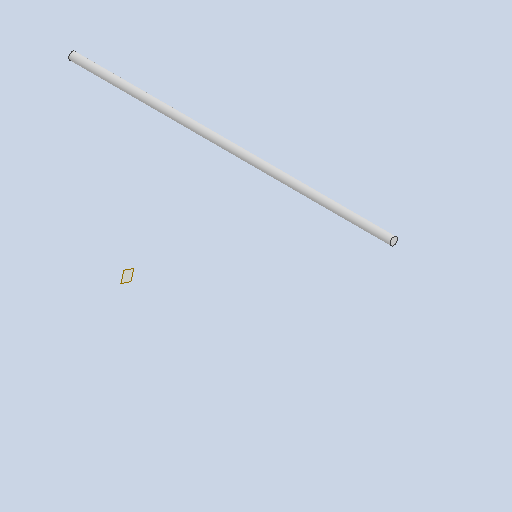
# Autodesk Inventor part: 12MM_X_AXIS_SHAFT
Saved by Autodesk Inventor 2025.2 (Build 292293000, 293)
## iProperties
Created: 2026-02-05
Part Number: 12MM_X_AXIS_SHAFT
Material: Generic
Document SubType Name: Modeling
Designer: composite
Density: 1 g/cm^3
Appearance: Default
Author: composite
Autodesk Inventor part; units mm, degrees
ref_plane "YZ Plane" through (0, 0, 0) normal (1, 0, 0) x (0, 1, 0)
ref_plane "XZ Plane" through (0, 0, 0) normal (0, 1, 0) x (-1, 0, 0)
ref_plane "XY Plane" through (0, 0, 0) normal (0, 0, 1) x (1, 0, 0)
sketch "Sketch1" plane through (0, 0, 0) normal (1, 0, 0) x (0, 1, 0)
  circle A0 centre (0, 0) radius 6
  dimension "d0" = 12
  constraints: 1 centre point, 1 coincident
  measures "d0" diameter of A0
extrude "Extrusion1" add sketch "Sketch1" along normal blind 10
sketch "Sketch2" plane through (0, 0, 0) normal (-1, 0, 0) x (0, 0, 1)
  circle A0 centre (0, 0) radius 6 projected
ref_plane "Work Plane1" through (-497, -256, -240) normal (-1, 0, 0) x (0, 0, 1)
ref_plane "Work Plane2" through (-697, -256, -240) normal (-1, 0, 0) x (0, 0, 1)
ref_plane "Work Plane3" through (-497, -256, -240) normal (-1, 0, 0) x (0, 0, 1)
ref_plane "Work Plane5" through (-481.5, -427.3957, -227.227) normal (1, 0, 0) x (0, 0.3162278, 0.9486833)
extrude "Extrusion3" add sketch "Sketch2" along normal up to surface (481.5 mm away)
sketch "Sketch3" plane through (-481.5, 0, 0) normal (-1, 0, 0) x (0, 0, 1)
  circle A0 centre (0, 0) radius 6 projected
  point P0 (0, 0)
ref_plane "Work Plane6" through (-500.5, -12.5, -12.5) normal (-1, 0, 0) x (0, 0, 1)
extrude "Extrusion4" add sketch "Sketch3" along normal up to surface (19 mm away)
body "Solid1"
